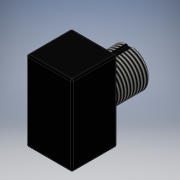
# Autodesk Inventor part: Toggle_Base
Saved by Autodesk Inventor 2016 (Build 200138000, 138)
## iProperties
Created: 2016-04-13
Part Number: Toggle_Base
Material: PC/ABS Plastic
Document SubType Name: Modeling
Designer: agmle
Density: 0.357273 g/cm^3
Appearance: Smooth - Black
Author: agmle
Autodesk Inventor part; units mm, degrees
ref_plane "YZ Plane" through (0, 0, 0) normal (1, 0, 0) x (0, 1, 0)
ref_plane "XZ Plane" through (0, 0, 0) normal (0, 1, 0) x (-1, 0, 0)
ref_plane "XY Plane" through (0, 0, 0) normal (0, 0, 1) x (1, 0, 0)
sketch "Sketch1" plane through (0, 0, 0) normal (0, 1, 0) x (-1, 0, 0)
  line L0 (7, 12.25) -> (-7, 12.25)
  line L1 (-7, 12.25) -> (-7, -12.25)
  line L2 (-7, -12.25) -> (7, -12.25)
  line L3 (7, -12.25) -> (7, 12.25)
  line L4 (7, 0) -> (-7, 0) construction
  point P0 (0, 0)
  point P1 (0, 0)
  dimension "d0" = 14
  dimension "d1" = 24.5
  constraints: 10 end point, 3 midpoint, 2 parallel, 1 coincident, 1 horizontal, 1 perpendicular
  measures "d0" distance of L0.start L0.end
  measures "d1" distance of L2.end L0.start
extrude "Extrusion1" add sketch "Sketch1" along normal blind 13.88
fillet "Fillet1" radius 0.5 12 edges at (7, 6.94, 12.25) (-7, 6.94, 12.25) (-7, 6.94, -12.25) (7, 6.94, -12.25) (7, 13.88, 0) (0, 13.88, -12.25) (-7, 13.88, 0) (0, 13.88, 12.25) (0, 0, 12.25) (7, 0, 0) (0, 0, -12.25) (-7, 0, 0)
sketch "Sketch2" plane through (0, 13.88, 0) normal (0, 1, 0) x (1, 0, 0)
  arc A0 (1, -5.8146) -> (-1, -5.8146) centre (0, 0) ccw
  circle A1 centre (0, 0) radius 3.94
  line L0 (1, -5.8146) -> (1, -5.0646)
  line L1 (1, -5.0646) -> (-1, -5.0646)
  line L2 (-1, -5.0646) -> (-1, -5.8146)
  line L3 (0, 0) -> (0, -5.0646) construction
  dimension "d5" = 11.8
  dimension "d8" = 7.88
  dimension "d9" = 0.75
  dimension "d10" = 2
  constraints: 8 end point, 2 centre point, 2 coincident, 2 perpendicular, 2 point on circle, 1 midpoint, 1 parallel
  measures "d5" diameter of A0
  measures "d8" diameter of A1
  measures "d9" distance of L1.end L2.end
  measures "d10" distance of L0.end L1.end
extrude "Extrusion3" add sketch "Sketch2" along normal blind 11.15
chamfer "Chamfer1" distance 0.5 angle 45 1 edges at (0, 25.03, -5.9)
thread "Thread1" size "M12x1" class "6g" standard "ANSI Metric M Profile" full length
body "Solid1"
